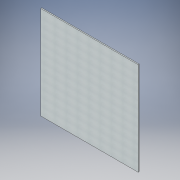
# Autodesk Inventor part: left_0_0
Saved by Autodesk Inventor 2019 (Build 230136000, 136)
## iProperties
Created: 2018-07-10
Part Number: left_0_0
Material: Generic
Document SubType Name: Modeling
Designer: User
Density: 1 g/cm^3
Appearance: Wood - Painted White
Author: User
Autodesk Inventor part; units mm, degrees
ref_plane "YZ Plane" through (0, 0, 0) normal (1, 0, 0) x (0, 1, 0)
ref_plane "XZ Plane" through (0, 0, 0) normal (0, 1, 0) x (-1, 0, 0)
ref_plane "XY Plane" through (0, 0, 0) normal (0, 0, 1) x (1, 0, 0)
sketch "Sketch1" plane through (0, 0, 0) normal (0, 0, 1) x (1, 0, 0)
  line L0 (-571.5, -546.1) -> (571.5, -546.1)
  line L1 (571.5, -546.1) -> (571.5, 546.1)
  line L2 (571.5, 546.1) -> (-571.5, 546.1)
  line L3 (-571.5, 546.1) -> (-571.5, -546.1)
  line L4 (-571.5, -546.1) -> (571.5, 546.1) construction
  line L5 (571.5, -546.1) -> (-571.5, 546.1) construction
  point P0 (0, 0)
  dimension "d0" = 1143
  dimension "d1" = 1092.2
  constraints: 12 end point, 2 midpoint, 2 parallel, 1 horizontal, 1 perpendicular
  measures "d0" distance of L1.end L2.end
  measures "d1" distance of L2.end L0.start
extrude "Extrusion1" add sketch "Sketch1" along normal blind 12.7
body "Solid1"
